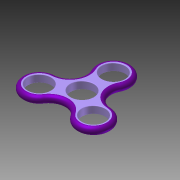
# Autodesk Inventor part: FidgetSpinnerBody
Saved by Autodesk Inventor 2011 SP2 (Build 150309200, 309)
## iProperties
Created: 2023-02-27
Part Number: FidgetSpinnerBody
Document SubType Name: Modeling
Designer: utilizator
Density: 1 g/cm^3
Author: utilizator
Autodesk Inventor part; units mm, degrees
ref_plane "YZ Plane" through (0, 0, 0) normal (1, 0, 0) x (0, 1, 0)
ref_plane "XZ Plane" through (0, 0, 0) normal (0, 1, 0) x (-1, 0, 0)
ref_plane "XY Plane" through (0, 0, 0) normal (0, 0, 1) x (1, 0, 0)
sketch "Sketch1" plane through (0, 0, 0) normal (0, 0, 1) x (1, 0, 0)
  circle A0 centre (0, 0) radius 11
  circle A1 centre (0, 30) radius 11
  circle A2 centre (0, 30) radius 16
  circle A3 centre (-25.9808, -15) radius 11
  circle A4 centre (-25.9808, -15) radius 16
  circle A5 centre (25.9808, -15) radius 11
  circle A6 centre (25.9808, -15) radius 16
  arc A7 (-26.8352, 0.9772) -> (-14.2638, 22.7514) centre (-27.6362, 15.9558) ccw
  arc A8 (12.5713, -23.7285) -> (-12.5713, -23.7285) centre (0, -31.9115) ccw
  arc A9 (14.2638, 22.7514) -> (26.8352, 0.9772) centre (27.6362, 15.9558) ccw
  dimension "d0" = 11
  dimension "d1" = 22
  dimension "d2" = 30
  dimension "d3" = 5
  dimension "d6" = 360
  dimension "d8" = 15
  dimension "d9" = 15
  dimension "d10" = 15
  constraints: 12 point on circle, 10 centre point, 6 tangent, 4 coincident, 1 vertical alignment, 13 other
  measures "d0" radius of A0
  measures "d1" diameter of A1
  measures "d2" distance of point (0, 0) A1.centre
  measures "d3" radial gap between concentric circles of A2 A1
  measures "d8" radius of A7
  measures "d9" radius of A8
  measures "d10" radius of A9
extrude "Extrusion1" add sketch "Sketch1" along normal blind 7
full round fillet "Fillet1" first side at (6.8143, 15.185, 7) centre faces at (-11.8514, -22.7167, 2.3333) second side at (6.8143, 15.185, 0)
fillet "Fillet2" radius 0.5 8 edges at (-36.9808, -15, 7) (-36.9808, -15, 0) (-11, 0, 7) (-11, 0, 0) (-11, 30, 7) (-11, 30, 0) (14.9808, -15, 7) (14.9808, -15, 0)
body "Solid1"
